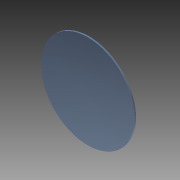
# Autodesk Inventor part: lente
Saved by Autodesk Inventor 2015 (Build 190159000, 159)
## iProperties
Created: 2015-03-17
Part Number: lente
Material: Genérico
Document SubType Name: Modeling
Designer: david_000
Density: 1 g/cm^3
Appearance: Valor por defecto
Author: david_000
Autodesk Inventor part; units mm, degrees
ref_plane "YZ Plane" through (0, 0, 0) normal (1, 0, 0) x (0, 1, 0)
ref_plane "XZ Plane" through (0, 0, 0) normal (0, 1, 0) x (-1, 0, 0)
ref_plane "XY Plane" through (0, 0, 0) normal (0, 0, 1) x (1, 0, 0)
sketch "Boceto1" plane through (0, 0, 0) normal (0, 0, 1) x (1, 0, 0)
  line L0 (0, 0) -> (63.5, 0)
  line L1 (63.5, 0) -> (63.5, 2)
  line L2 (0, 0) -> (0, 6)
  arc A0 (63.5, 2) -> (0, 6) centre (0, -500.0313) ccw
  line L3 (0, 0) -> (0, -10000)
  arc A1 (63.5, 0) -> (0, 4.0159) centre (0, -500.0313) ccw
  dimension "d0" = 63.5
  dimension "d1" = 2
  dimension "d2" = 6
  dimension "d3" = 10000
  constraints: 8 end point, 4 point on circle, 2 centre point, 2 point on line, 2 vertical, 1 coincident, 1 horizontal, 1 perpendicular
  measures "d0" distance of L0.start L0.end
  measures "d1" distance of L0.end L1.end
  measures "d2" distance of L2.end L0.start
  measures "d3" distance of L0.start L3.end
revolve "Revolución1" add sketch "Boceto1" angle 360 about axis through (0, 0, 0) along (0, 1, 0) contours A1 L2 A0 L1
